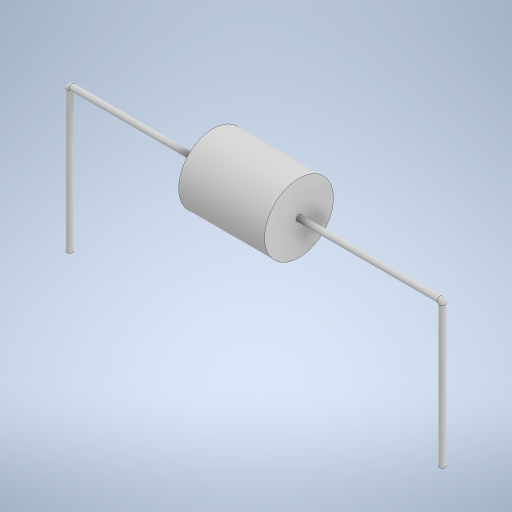
# Autodesk Inventor part: KC139
Saved by Autodesk Inventor 2024 (Build 280153000, 153)
## iProperties
Created: 2023-12-19
Part Number: KC139
Material: Generic
Document SubType Name: Sheet Metal
Designer: user
Density: 1 g/cm^3
Sheet Metal Rule: Default
Appearance: Default
Author: user
Autodesk Inventor part; units mm, degrees
ref_plane "YZ Plane" through (0, 0, 0) normal (1, 0, 0) x (0, 1, 0)
sketch "Sketch1" plane through (0, 0, 0) normal (0, 0, 1) x (1, 0, 0)
  line L0 (0, 0) -> (7.5, 0)
  line L1 (7.5, 0) -> (7.5, 3)
  line L2 (7.5, 3) -> (0, 3)
  line L3 (0, 3) -> (0, 0)
  dimension "d0" = 7.5
  dimension "d1" = 3
  constraints: 8 end point, 2 parallel, 1 horizontal, 1 perpendicular
  measures "d0" distance of L2.end L1.end
  measures "d1" distance of L1.end L0.end
revolve "Revolution1" add sketch "Sketch1" angle 360 about axis through (0, 0, 0) along (1, 0, 0)
sketch "Sketch2" plane through (0, 0, 0) normal (0, 0, 1) x (1, 0, 0)
  line L0 (7.5, -3) -> (7.5, 3) projected
  line L1 (7.5, 0) -> (19.8, 0)
  line L2 (20, -0.2) -> (20, -12.5)
  line L3 (0, 0) -> (-12.3, 0)
  line L4 (-12.5, -0.2) -> (-12.5, -12.5)
  arc A0 (-12.3, 0) -> (-12.5, -0.2) centre (-12.3, -0.2) ccw
  arc A1 (20, -0.2) -> (19.8, 0) centre (19.8, -0.2) ccw
  point P0 (20, 0)
  point P1 (-12.5, 0)
  dimension "d3" = 12.5
  dimension "d4" = 12.5
  dimension "d5" = 12.5
  dimension "d6" = 12.5
  dimension "d7" = 0.2
  constraints: 8 end point, 4 point on circle, 4 point on line, 4 tangent, 2 centre point, 2 horizontal, 2 perpendicular, 1 equal radius, 1 midpoint
  measures "d3" distance of L1.start point (20, 0)
  measures "d4" distance of point (20, 0) L2.end
  measures "d5" distance of L3.start point (-12.5, 0)
  measures "d6" distance of point (-12.5, 0) L4.end
  measures "d7" radius of A0
ref_plane "Work Plane1" through (7.5, 0, 0) normal (1, 0, 0) x (0, 0, -1)
ref_plane "Work Plane2" through (0, 0, 0) normal (-1, 0, 0) x (0, 0, 1)
sketch "Sketch3" plane through (7.5, 0, 0) normal (1, 0, 0) x (0, 0, -1)
  circle A0 centre (0, 0) radius 0.25
  dimension "d10" = 0.5
  constraints: 1 centre point, 1 coincident
  measures "d10" diameter of A0
sketch "Sketch4" plane through (0, 0, 0) normal (-1, 0, 0) x (0, 0, 1)
  circle A0 centre (0, 0) radius 0.25
  dimension "d11" = 0.5
  constraints: 1 centre point, 1 coincident
  measures "d11" diameter of A0
sweep "Sweep1" add profiles "Sketch4" path "Sketch2" path curves L3 A0 L4
sweep "Sweep2" add profiles "Sketch3" path "Sketch2" path curves L1 A1 L2
equation "\"BendRadius\" = Thickness"
equation "\"BendReliefWidth\" = Thickness"
equation "\"BendReliefDepth\" = 0.5 * Thickness"
equation "\"CornerReliefSize\" = 4 * Thickness"
equation "\"MinimumRemnant\" = 2 * Thickness"
equation "\"TransitionRadius\" = BendRadius"
equation "\"JacobiRadiusSize\" = BendRadius"
equation "\"GapSize\" = Thickness"
equation "\"Thickness\" = 3.048"
body "Solid1"
